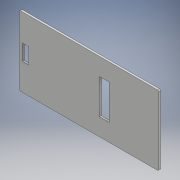
# Autodesk Inventor part: AtasFix
Saved by Autodesk Inventor 2017 (Build 210142000, 142)
## iProperties
Created: 2019-05-10
Part Number: AtasFix
Material: Generic
Document SubType Name: Modeling
Designer: Faiz
Density: 1 g/cm^3
Appearance: Default
Author: Faiz
Autodesk Inventor part; units mm, degrees
ref_plane "YZ Plane" through (0, 0, 0) normal (1, 0, 0) x (0, 1, 0)
ref_plane "XZ Plane" through (0, 0, 0) normal (0, 1, 0) x (-1, 0, 0)
ref_plane "XY Plane" through (0, 0, 0) normal (0, 0, 1) x (1, 0, 0)
sketch "Sketch1" plane through (0, 0, 0) normal (0, 1, 0) x (-1, 0, 0)
  line L0 (108, 55) -> (-108, 55)
  line L1 (-110, 53) -> (-110, -53)
  line L2 (-108, -55) -> (108, -55)
  line L3 (110, -53) -> (110, 53)
  arc A0 (110, 53) -> (108, 55) centre (108, 53) ccw
  arc A1 (108, -55) -> (110, -53) centre (108, -53) ccw
  arc A2 (-110, -53) -> (-108, -55) centre (-108, -53) ccw
  arc A3 (-108, 55) -> (-110, 53) centre (-108, 53) ccw
  point P0 (0, 0)
  constraints: 8 end point, 8 point on circle, 8 tangent, 4 centre point, 3 equal radius, 2 parallel, 1 horizontal, 1 perpendicular
extrude "Extrusion1" add sketch "Sketch1" along normal mid plane 3
sketch "Sketch2" plane through (0, 1.5, 0) normal (0, 1, 0) x (1, 0, 0)
  line L0 (12.1921, -50) -> (92.1921, -50)
  line L1 (92.1921, -50) -> (92.1921, 50)
  line L2 (92.1921, 50) -> (12.1921, 50)
  line L3 (12.1921, 50) -> (12.1921, -50)
  line L4 (-95.242, 12.5) -> (-105.242, 12.5)
  line L5 (-105.242, 12.5) -> (-105.242, -12.5)
  line L6 (-105.242, -12.5) -> (-95.242, -12.5)
  line L7 (-95.242, -12.5) -> (-95.242, 12.5)
  circle A0 centre (5.4677, -30.1554) radius 1.5
  line L8 (0, 0) -> (5.4677, 0)
  circle A1 centre (5.4677, 30.1554) radius 1.5
  line L9 (-4.7214, 27.5) -> (-89.7214, 27.5)
  line L10 (-89.7214, 27.5) -> (-89.7214, -27.5)
  line L11 (-89.7214, -27.5) -> (-4.7214, -27.5)
  line L12 (-4.7214, -27.5) -> (-4.7214, 27.5)
  line L13 (16.5249, 27.5) -> (31.5249, 27.5)
  line L14 (31.5249, 27.5) -> (31.5249, -27.5)
  line L15 (31.5249, -27.5) -> (16.5249, -27.5)
  line L16 (16.5249, -27.5) -> (16.5249, 27.5)
  point P0 (52.1921, 0)
  constraints: 34 end point, 8 parallel, 5 horizontal, 4 perpendicular, 2 centre point, 1 symmetric about line, 1 other
extrude "Extrusion2" cut sketch "Sketch2" against normal blind 3 contours L7 L6 L5 L4 | L13 L14 L15 L16
sketch "Sketch3" plane through (0, 1.5, 0) normal (0, 1, 0) x (1, 0, 0)
  point P0 (0, 0)
body "Solid1"
